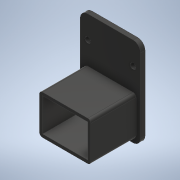
# Autodesk Inventor part: ButtonBox
Saved by Autodesk Inventor 2020.2 (Build 242310000, 310)
## iProperties
Created: 2019-02-15
Part Number: ButtonBox
Material: Generic
Document SubType Name: Modeling
Designer: JK
Density: 1 g/cm^3
Appearance: Smooth - Black
Author: JK
Autodesk Inventor part; units mm, degrees
ref_plane "YZ Plane" through (0, 0, 0) normal (1, 0, 0) x (0, 1, 0)
ref_plane "XZ Plane" through (0, 0, 0) normal (0, 1, 0) x (-1, 0, 0)
ref_plane "XY Plane" through (0, 0, 0) normal (0, 0, 1) x (1, 0, 0)
sketch "Sketch1" plane through (0, 0, 0) normal (0, 1, 0) x (-1, 0, 0)
  line L0 (-20, 24.5) -> (20, 24.5)
  line L1 (20, 24.5) -> (20, -24.5)
  line L2 (20, -24.5) -> (-20, -24.5)
  line L3 (-20, -24.5) -> (-20, 24.5)
  line L4 (-20, 24.5) -> (20, -24.5) construction
  line L5 (20, 24.5) -> (-20, -24.5) construction
  circle A0 centre (15, 19.5) radius 1.9
  circle A1 centre (-15, 19.5) radius 1.9
  line L6 (15, 2.5) -> (-15, 2.5)
  line L7 (-15, 2.5) -> (-15, -19.5)
  line L8 (-15, -19.5) -> (15, -19.5)
  line L9 (15, -19.5) -> (15, 2.5)
  line L10 (15, 2.5) -> (-15, -19.5) construction
  line L11 (-15, 2.5) -> (15, -19.5) construction
  point P0 (0, 0)
  point P1 (15, 17.5)
  point P2 (-15, 17.5)
  point P3 (0, -8.5)
  point P4 (0, -8.5)
  point P5 (0, 0)
  dimension "d0" = 30
  dimension "d1" = 3.8
  dimension "d4" = 5
  dimension "d5" = 15
  dimension "d6" = 22
  dimension "d7" = 30
  dimension "d9" = 49
  dimension "d12" = 40
  dimension "d21" = 22
  constraints: 24 end point, 6 midpoint, 4 parallel, 2 centre point, 2 horizontal, 2 perpendicular, 1 equal radius, 1 horizontal alignment, 1 vertical alignment
  measures "d0" distance of A1.centre A0.centre
  measures "d1" diameter of A0
  measures "d4" distance from line of L0 A0.centre
  measures "d5" horizontal distance of point (0, 0) A0.centre
  measures "d6" distance of L6.end L7.end
  measures "d7" distance of L7.end L8.end
  measures "d9" distance of L0.end L1.end
  measures "d12" distance of L0.start L0.end
  measures "d21" distance between parallel lines of L0 L6
extrude "Extrusion1" add sketch "Sketch1" along normal blind 3
sketch "Sketch2" plane through (0, 0, 0) normal (0, -1, 0) x (1, 0, 0)
  point P0 (0, 0)
sketch "Sketch3" plane through (0, 0, 0) normal (0, -1, 0) x (1, 0, 0)
  line L0 (17, -21.5) -> (-17, -21.5)
  line L1 (-17, -21.5) -> (-17, 4.5)
  line L2 (-17, 4.5) -> (17, 4.5)
  line L3 (17, 4.5) -> (17, -21.5)
  line L4 (17, -21.5) -> (-17, 4.5) construction
  line L5 (-17, -21.5) -> (17, 4.5) construction
  line L6 (-15, -19.5) -> (-15, 2.5) projected
  line L7 (15, 2.5) -> (15, -19.5) projected
  line L8 (15, -19.5) -> (-15, -19.5) projected
  line L9 (-15, 2.5) -> (15, 2.5) projected
  line L10 (15, 2.5) -> (-15, 2.5) projected
  line L11 (15, -19.5) -> (-15, -19.5)
  line L12 (-15, -19.5) -> (-15, 2.5)
  line L13 (-15, 2.5) -> (15, 2.5)
  line L14 (15, 2.5) -> (15, -19.5)
  line L15 (15, -19.5) -> (-15, 2.5) construction
  line L16 (-15, -19.5) -> (15, 2.5) construction
  point P0 (0, 0)
  point P1 (0, -8.5)
  point P2 (0, -8.5)
  dimension "d13" = 2
  dimension "d14" = 2
  dimension "d15" = 2
  dimension "d16" = 2
  constraints: 24 end point, 6 midpoint, 4 parallel, 2 horizontal, 2 perpendicular
  measures "d13" distance between parallel lines of L6 L1
  measures "d14" distance between parallel lines of L7 L3
  measures "d15" distance between parallel lines of L8 L0
  measures "d16" distance between parallel lines of L2 L9
extrude "Extrusion2" add sketch "Sketch3" along normal blind 30
fillet "Fillet1" radius 5 4 edges at (-20, 1.5, -24.5) (-20, 1.5, 24.5) (20, 1.5, 24.5) (20, 1.5, -24.5)
fillet "Fillet2" radius 2 4 edges at (-17, -15, -21.5) (17, -15, 4.5) (-17, -15, 4.5) (17, -15, -21.5)
sketch "Sketch4" plane through (0, 3, 0) normal (0, 1, 0) x (1, 0, 0)
  line L0 (-15, -24.5) -> (15, -24.5) projected
  arc A0 (15, -24.5) -> (20, -19.5) centre (15, -19.5) ccw projected
  arc A1 (-20, -19.5) -> (-15, -24.5) centre (-15, -19.5) ccw projected
  line L1 (20, -19.5) -> (-20, -19.5)
  line L2 (-20, -19.5) -> (-20, -34.5)
  line L3 (-20, -34.5) -> (20, -34.5)
  line L4 (20, -34.5) -> (20, -19.5)
  point P0 (0, 0)
  dimension "d22" = 15
  constraints: 8 end point, 2 parallel, 1 horizontal, 1 perpendicular
  measures "d22" distance of L3.end L1.start
extrude "Extrusion3" add sketch "Sketch4" against normal up to surface (3 mm away) contours L0 A0 L4 L3 L2 A1
fillet "Fillet3" radius 5 2 edges at (20, 1.5, 34.5) (-20, 1.5, 34.5)
body "Solid1"
